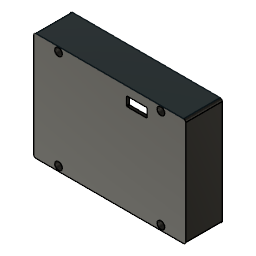
Fibonacci Back (Autodesk Fusion 360 design; units mm, degrees)
Autodesk Fusion 360 part; units mm, degrees
sketch "Sketch1" plane through (0, 0, 0) normal (0, 1, 0) x (1, 0, 0)
  arc A0 (-114.2414, 36.1703) -> (-116.2414, 34.1703) centre (-114.2414, 34.1703) ccw
  arc A1 (-114.2414, 36.1703) -> (-116.2414, 34.1703) centre (-114.2414, 34.1703) ccw
  arc A2 (-13.2414, -38.8297) -> (-11.2414, -36.8297) centre (-13.2414, -36.8297) ccw
  arc A3 (-116.2414, -36.8297) -> (-114.2414, -38.8297) centre (-114.2414, -36.8297) ccw
  arc A4 (-116.2414, -36.8297) -> (-114.2414, -38.8297) centre (-114.2414, -36.8297) ccw
  arc A5 (-13.2414, -38.8297) -> (-11.2414, -36.8297) centre (-13.2414, -36.8297) ccw
  circle A6 centre (-98.7415, -35.0863) radius 1.55
  circle A7 centre (-98.7415, 32.427) radius 1.55
  line L0 (-11.2414, -36.8297) -> (-11.2414, 34.1703)
  circle A8 centre (-28.7414, -35.0863) radius 1.55
  arc A9 (-11.2414, 34.1703) -> (-13.2414, 36.1703) centre (-13.2414, 34.1703) ccw
  arc A10 (-11.2414, 34.1703) -> (-13.2414, 36.1703) centre (-13.2414, 34.1703) ccw
  circle A11 centre (-28.7414, 32.427) radius 1.55
  line L1 (-116.2414, -36.8297) -> (-116.2414, 34.1703)
  line L2 (-13.2414, 36.1703) -> (-114.2414, 36.1703)
  line L3 (-114.2414, 36.1703) -> (-13.2414, 36.1703)
  line L4 (-114.2414, -38.8297) -> (-13.2414, -38.8297)
  line L5 (-116.2414, 34.1703) -> (-116.2414, -36.8297)
  line L6 (-11.2414, 34.1703) -> (-11.2414, -36.8297)
  line L7 (-13.2414, -38.8297) -> (-114.2414, -38.8297)
  line L8 (-12.7414, -36.8297) -> (-12.7414, 34.1703)
  arc A12 (-12.7414, 34.1703) -> (-13.2414, 34.6703) centre (-13.2414, 34.1703) ccw
  line L9 (-13.2414, 34.6703) -> (-114.2414, 34.6703)
  arc A13 (-114.2414, 34.6703) -> (-114.7414, 34.1703) centre (-114.2414, 34.1703) ccw
  line L10 (-114.7414, 34.1703) -> (-114.7414, -36.8297)
  arc A14 (-114.7414, -36.8297) -> (-114.2414, -37.3297) centre (-114.2414, -36.8297) ccw
  line L11 (-114.2414, -37.3297) -> (-13.2414, -37.3297)
  arc A15 (-13.2414, -37.3297) -> (-12.7414, -36.8297) centre (-13.2414, -36.8297) ccw
  circle A16 centre (-98.7415, -35.0863) radius 2.6
  circle A17 centre (-28.7414, -35.0863) radius 2.6
  circle A18 centre (-98.7415, 32.427) radius 2.6
  circle A19 centre (-28.7414, 32.427) radius 2.6
  circle A20 centre (-98.7415, -35.0863) radius 1.9
  circle A21 centre (-28.7414, -35.0863) radius 1.9
  circle A22 centre (-98.7415, 32.427) radius 1.9
  circle A23 centre (-28.7414, 32.427) radius 1.9
  line L12 (-11.7414, -36.8297) -> (-11.7414, 34.1703)
  arc A24 (-11.7414, 34.1703) -> (-13.2414, 35.6703) centre (-13.2414, 34.1703) ccw
  line L13 (-13.2414, 35.6703) -> (-114.2414, 35.6703)
  arc A25 (-114.2414, 35.6703) -> (-115.7414, 34.1703) centre (-114.2414, 34.1703) ccw
  line L14 (-115.7414, 34.1703) -> (-115.7414, -36.8297)
  arc A26 (-115.7414, -36.8297) -> (-114.2414, -38.3297) centre (-114.2414, -36.8297) ccw
  line L15 (-114.2414, -38.3297) -> (-13.2414, -38.3297)
  arc A27 (-13.2414, -38.3297) -> (-11.7414, -36.8297) centre (-13.2414, -36.8297) ccw
  line L16 (-38.2137, -26.6593) -> (-38.2137, -31.8593)
  line L17 (-38.7137, -32.3593) -> (-51.7137, -32.3593)
  arc A28 (-52.2137, -31.8593) -> (-51.7137, -32.3593) centre (-51.7137, -31.8593) ccw
  line L18 (-52.2137, -31.8593) -> (-52.2137, -26.6593)
  arc A29 (-38.2137, -26.6593) -> (-38.7137, -26.1593) centre (-38.7137, -26.6593) ccw
  line L19 (-51.7137, -26.1593) -> (-38.7137, -26.1593)
  arc A30 (-38.7137, -32.3593) -> (-38.2137, -31.8593) centre (-38.7137, -31.8593) ccw
  arc A31 (-51.7137, -26.1593) -> (-52.2137, -26.6593) centre (-51.7137, -26.6593) ccw
  point P0 (-38.2137, -32.3593)
  point P1 (-52.2137, -32.3593)
  point P2 (-52.2137, -26.1593)
  dimension "d1" = -1.5
  dimension "d16" = 5.2
  dimension "d17" = 5.2
  dimension "d18" = 5.2
  dimension "d19" = 5.2
  dimension "d22" = 3.8
  dimension "d23" = 3.8
  dimension "d24" = 3.8
  dimension "d25" = 3.8
  dimension "d28" = -0.5
  dimension "d31" = 6.2
  dimension "d32" = 14
  dimension "d33" = 0.5
  dimension "d34" = 0.5
  dimension "d35" = 0.5
  constraint concentric A6 A16
  constraint concentric A8 A17
  constraint concentric A7 A18
  constraint concentric A11 A19
  constraint concentric A16 A20
  constraint concentric A8 A21
  constraint concentric A7 A22
  constraint concentric A11 A23
  constraint horizontal L19
  constraint vertical L16
  constraint horizontal L17
  constraint vertical L18
  constraint coincident P1 L17
  constraint coincident P1 L18
  constraint tangent L17 A28
  constraint tangent A28 L18
  constraint coincident P0 L17
  constraint coincident P0 L16
  constraint tangent L17 A30
  constraint tangent L16 A30
  constraint tangent A29 L19
  constraint tangent L16 A29
  constraint equal A29 A30
  constraint coincident P2 L18
  constraint coincident P2 L19
  constraint tangent L18 A31
  constraint tangent L19 A31
  measures "d16" diameter of A16
  measures "d17" diameter of A17
  measures "d18" diameter of A18
  measures "d19" diameter of A19
  measures "d22" diameter of A20
  measures "d23" diameter of A21
  measures "d24" diameter of A22
  measures "d25" diameter of A23
  measures "d31" distance of P1 P2
  measures "d32" distance of P0 P1
  measures "d33" radius of A28
  measures "d34" radius of A30
  measures "d35" radius of A31
extrude "Extrude1" add sketch "Sketch1" along normal blind 1.9 contours A0 A1 A2 A3 A4 A5 L0 A9 A10 L1 L2 L3 L4 L5 L6 L7 | L8 A12 L9 A13 L10 A14 L11 A15 A16 A17 A18 A19 | L11 A17 | L11 A17 | L9 A19 | L9 A19 | L11 A16 | L11 A16 | L9 A18 | L9 A18 | A20 | A21 | A22 | A23 | L12 A24 L13 A25 L14 A26 L15 A27 | L16 L17 A28 L18 A29 L19 A30 A31
extrude "Extrude2" add sketch "Sketch1" along normal blind 25 contours A0 A1 A2 A3 A4 A5 L0 A9 A10 L1 L2 L3 L4 L5 L6 L7 | L11 A17 | L9 A19 | L11 A16 | L9 A18 | L12 A24 L13 A25 L14 A26 L15 A27 picked at (-28.4059, -37.381) picked at (-28.6269, 34.8843) picked at (-98.406, -37.381) picked at (-98.9586, 34.8329)
sketch "Sketch2" plane through (0, 1.9, 0) normal (0, 1, 0) x (-1, 0, 0)
  line L0 (12.7414, 36.8297) -> (12.7414, -34.1703)
  arc A0 (12.7414, -34.1703) -> (13.2414, -34.6703) centre (13.2414, -34.1703) ccw
  line L1 (13.2414, -34.6703) -> (114.2414, -34.6703)
  arc A1 (114.2414, -34.6703) -> (114.7414, -34.1703) centre (114.2414, -34.1703) ccw
  line L2 (114.7414, -34.1703) -> (114.7414, 36.8297)
  arc A2 (114.7414, 36.8297) -> (114.2414, 37.3297) centre (114.2414, 36.8297) ccw
  line L3 (114.2414, 37.3297) -> (13.2414, 37.3297)
  arc A3 (13.2414, 37.3297) -> (12.7414, 36.8297) centre (13.2414, 36.8297) ccw
  circle A4 centre (98.7415, 35.0863) radius 1.55
  circle A5 centre (98.7415, -32.427) radius 1.55
  circle A6 centre (28.7414, -32.427) radius 1.55
  circle A7 centre (28.7414, 35.0863) radius 1.55
  line L4 (32.2414, 38.5863) -> (25.2414, 38.5863)
  line L5 (25.2414, 38.5863) -> (25.2414, 31.5863)
  line L6 (25.2414, 31.5863) -> (32.2414, 31.5863)
  line L7 (32.2414, 31.5863) -> (32.2414, 38.5863)
  line L8 (32.2414, 38.5863) -> (25.2414, 31.5863) construction
  line L9 (25.2414, 38.5863) -> (32.2414, 31.5863) construction
  line L10 (102.2415, 38.5863) -> (95.2415, 38.5863)
  line L11 (95.2415, 38.5863) -> (95.2415, 31.5863)
  line L12 (95.2415, 31.5863) -> (102.2415, 31.5863)
  line L13 (102.2415, 31.5863) -> (102.2415, 38.5863)
  line L14 (102.2415, 38.5863) -> (95.2415, 31.5863) construction
  line L15 (95.2415, 38.5863) -> (102.2415, 31.5863) construction
  line L16 (32.2414, -28.927) -> (25.2414, -28.927)
  line L17 (25.2414, -28.927) -> (25.2414, -35.927)
  line L18 (25.2414, -35.927) -> (32.2414, -35.927)
  line L19 (32.2414, -35.927) -> (32.2414, -28.927)
  line L20 (32.2414, -28.927) -> (25.2414, -35.927) construction
  line L21 (25.2414, -28.927) -> (32.2414, -35.927) construction
  line L22 (102.2415, -28.927) -> (95.2415, -28.927)
  line L23 (95.2415, -28.927) -> (95.2415, -35.927)
  line L24 (95.2415, -35.927) -> (102.2415, -35.927)
  line L25 (102.2415, -35.927) -> (102.2415, -28.927)
  line L26 (102.2415, -28.927) -> (95.2415, -35.927) construction
  line L27 (95.2415, -28.927) -> (102.2415, -35.927) construction
  point P0 (28.7414, 35.0863)
  point P1 (98.7415, 35.0863)
  point P2 (28.7414, -32.427)
  point P3 (98.7415, -32.427)
  dimension "d6" = 7
  dimension "d7" = 7
  dimension "d8" = 7
  dimension "d9" = 7
  dimension "d10" = 7
  dimension "d11" = 7
  dimension "d12" = 7
  dimension "d13" = 7
  constraint horizontal L4
  constraint perpendicular L4 L5
  constraint parallel L4 L6
  constraint parallel L5 L7
  constraint coincident L8 P0
  constraint coincident L9 P0
  constraint coincident P0 A7.centre
  constraint horizontal L10
  constraint perpendicular L10 L11
  constraint parallel L10 L12
  constraint parallel L11 L13
  constraint coincident L14 P1
  constraint coincident L15 P1
  constraint coincident P1 A4.centre
  constraint horizontal L16
  constraint perpendicular L16 L17
  constraint parallel L16 L18
  constraint parallel L17 L19
  constraint coincident L20 P2
  constraint coincident L21 P2
  constraint coincident P2 A6.centre
  constraint horizontal L22
  constraint perpendicular L22 L23
  constraint parallel L22 L24
  constraint parallel L23 L25
  constraint coincident L26 P3
  constraint coincident L27 P3
  constraint coincident P3 A5.centre
  measures "d6" distance of L5.end L6.end
  measures "d7" distance of L4.end L5.end
  measures "d8" distance of L11.end L12.end
  measures "d9" distance of L10.end L11.end
  measures "d10" distance of L17.end L18.end
  measures "d11" distance of L16.end L17.end
  measures "d12" distance of L23.end L24.end
  measures "d13" distance of L22.end L23.end
extrude "Extrude3" add sketch "Sketch2" along normal blind 17.2 contours L3 L5 L6 L7 | L1 L16 L17 L19 | L3 L11 L12 L13 | L1 L22 L23 L25
extrude "Extrude4" cut sketch "Sketch1" along normal blind 5 contours L11 A17 | L11 A17 | L9 A19 | L9 A19 | L11 A16 | L11 A16 | L9 A18 | L9 A18 | A20 | A21 | A22 | A23
extrude "Extrude5" cut sketch "Sketch1" along normal blind 38 contours A20 | A21 | A22 | A23
extrude "Extrude6" cut sketch "Sketch1" along normal blind 69 contours A0 A1 A2 A3 A4 A5 L0 A9 A10 L1 L2 L3 L4 L5 L6 L7
extrude "Extrude7" cut sketch "Sketch1" along normal blind 24 contours L16 L17 A28 L18 A29 L19 A30 A31
sketch "Sketch3" plane through (0, 0, 38.3297) normal (0, 0, 1) x (-1, 0, 0)
  line L0 (13.2414, -25) -> (114.2414, -25)
  line L1 (114.2414, -25) -> (114.2414, 0)
  line L2 (114.2414, 0) -> (13.2414, 0)
  line L3 (13.2414, 0) -> (13.2414, -25)
equation "d14 = 19.00 mm - 1.8 mm"
